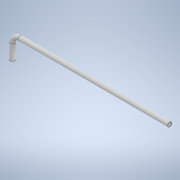
# Autodesk Inventor part: Pipe
Saved by Autodesk Inventor 2020.3 (Build 243373000, 373)
## iProperties
Created: 2020-11-11
Part Number: Pipe
Material: Generic
Document SubType Name: Modeling
Designer: Naude Conradie
Density: 1 g/cm^3
Appearance: Default
Author: Naude Conradie
Autodesk Inventor part; units mm, degrees
ref_plane "YZ Plane" through (0, 0, 0) normal (1, 0, 0) x (0, 1, 0)
ref_plane "XZ Plane" through (0, 0, 0) normal (0, 1, 0) x (-1, 0, 0)
ref_plane "XY Plane" through (0, 0, 0) normal (0, 0, 1) x (1, 0, 0)
sketch "Sketch1" plane through (0, 0, 0) normal (0, 1, 0) x (-1, 0, 0)
  circle A0 centre (0, 0) radius 2
  circle A1 centre (0, 0) radius 3
  dimension "d0" = 4
  dimension "d1" = 6
  constraints: 2 centre point, 2 coincident
  measures "d0" diameter of A0
  measures "d1" diameter of A1
extrude "Extrusion1" add sketch "Sketch1" along normal blind 20
sketch "Sketch2" plane through (0, 20, 0) normal (0, 1, 0) x (1, 0, 0)
  circle A0 centre (0, 0) radius 3 projected
  circle A1 centre (0, 0) radius 2 projected
  line L0 (10, -5) -> (10, 5)
  dimension "d4" = 10
  dimension "d5" = 5
  dimension "d6" = 10
  constraints: 2 end point, 1 vertical
  measures "d4" distance of L0.start L0.end
  measures "d5" vertical distance of L0.start point (0, 0)
  measures "d6" distance from line of L0 point (0, 0)
revolve "Revolution1" add sketch "Sketch2" angle 90 about axis through (10, 20, 5) along (0, 0, -1)
sketch "Sketch3" plane through (10, 30, 0) normal (1, 0, 0) x (0, 0, -1)
  circle A0 centre (0, 0) radius 3 projected
  circle A1 centre (0, 0) radius 2 projected
  point P0 (0, -30)
extrude "Extrusion2" add sketch "Sketch3" along normal blind 200
body "Solid1"
